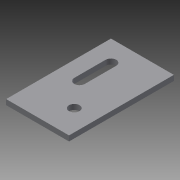
# Autodesk Inventor part: 8.2 Q1
Saved by Autodesk Inventor 2015 (Build 190159000, 159)
## iProperties
Created: 2018-04-11
Part Number: 8.2 Q1
Material: Generic
Document SubType Name: Modeling
Designer: Administrator
Density: 1 g/cm^3
Appearance: Default
Mass: 7.09626 g
Surface Area: 53.6289 cm^2
Volume: 7.09626 cm^3
Author: Administrator
Autodesk Inventor part; units mm, degrees
ref_plane "YZ Plane" through (0, 0, 0) normal (1, 0, 0) x (0, 1, 0)
ref_plane "XZ Plane" through (0, 0, 0) normal (0, 1, 0) x (-1, 0, 0)
ref_plane "XY Plane" through (0, 0, 0) normal (0, 0, 1) x (1, 0, 0)
sketch "Sketch1" plane through (0, 0, 0) normal (0, 1, 0) x (-1, 0, 0)
  line L0 (0, -63.5) -> (38.1, -63.5)
  line L1 (38.1, -63.5) -> (38.1, 0)
  line L2 (38.1, 0) -> (0, 0)
  line L3 (0, 0) -> (0, -63.5)
  line L4 (28.575, -31.75) -> (28.575, -50.8)
  line L5 (22.225, -50.8) -> (22.225, -31.75)
  arc A0 (28.575, -31.75) -> (22.225, -31.75) centre (25.4, -31.75) ccw
  arc A1 (22.225, -50.8) -> (28.575, -50.8) centre (25.4, -50.8) ccw
  circle A2 centre (12.7, -15.875) radius 3.175
  dimension "d0" = 38.1
  dimension "d2" = 63.5
  dimension "d3" = 19.05
  dimension "d4" = 50.8
  dimension "d5" = 12.7
  dimension "d6" = 15.875
  dimension "d7" = 25.4
  dimension "d10" = 3.175
  dimension "d11" = 3.175
  dimension "d12" = 6.35
  constraints: 12 end point, 4 point on circle, 4 tangent, 3 centre point, 3 perpendicular, 1 horizontal, 1 vertical
  measures "d0" distance of L0.start L0.end
  measures "d2" distance of L0.end L1.end
  measures "d3" distance of A1.centre A0.centre
  measures "d4" distance from line of A1.centre L2
  measures "d5" distance from line of A1.centre L1
  measures "d6" distance from line of A2.centre L2
  measures "d7" distance from line of A2.centre L1
  measures "d10" radius of A1
  measures "d11" radius of A0
  measures "d12" diameter of A2
extrude "Extrusion1" add sketch "Sketch1" along normal blind 3.175
equation "\"d2\" = 1.66667 * d0"
equation "\"d3\" = 0.5 * d0"
equation "\"d4\" = 0.8 * d2"
equation "\"d5\" = 0.333333 * d0"
equation "\"d6\" = 0.25 * d2"
equation "\"d7\" = 0.666667 * d0"
equation "\"d10\" = d8"
equation "\"d11\" = d8"
equation "\"d12\" = 2 * d8"
equation "\"d8\" = 0.05 * d2"
body "Solid1"
